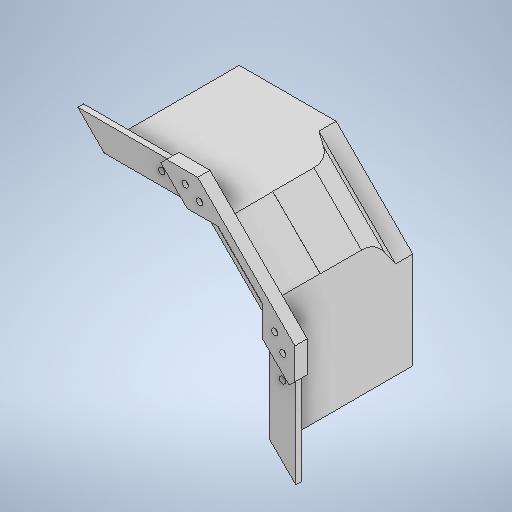
# Autodesk Inventor part: KimiBottomCover
Saved by Autodesk Inventor 2025.1 (Build 291241000, 241)
## iProperties
Created: 2026-05-07
Part Number: KimiBottomCover
Material: Generic
Document SubType Name: Modeling
Designer: User
Density: 1 g/cm^3
Appearance: Default
Author: User
## iProperties of the stored document KimiBottomCover_3DPrint.ipt
Created: 2026-05-07
Part Number: KimiBottomCover_3DPrint
Material: Generic
Document SubType Name: Modeling
Designer: User
Density: 1 g/cm^3
Appearance: Default
Author: User
Autodesk Inventor part; units mm, degrees
ref_plane "YZ Plane" through (0, 0, 0) normal (1, 0, 0) x (0, 1, 0)
ref_plane "XZ Plane" through (0, 0, 0) normal (0, 1, 0) x (-1, 0, 0)
ref_plane "XY Plane" through (0, 0, 0) normal (0, 0, 1) x (1, 0, 0)
sketch "Sketch1" plane through (0, 0, 0) normal (0, 0, 1) x (1, 0, 0)
  circle A0 centre (-3.4009, 1.926) radius 1.5 projected
  circle A1 centre (3.4009, -1.926) radius 1.5 projected
  circle A2 centre (38.7849, -37.31) radius 1.5 projected
  circle A3 centre (42.6369, -44.1118) radius 1.5 projected
  circle A4 centre (-3.4009, 1.926) radius 1.5 projected
  circle A5 centre (3.4009, -1.926) radius 1.5 projected
  line L0 (-12.5711, 5.5) -> (-1.5711, -5.5) projected
  line L1 (-1.5711, -5.5) -> (12.5711, -5.5) projected
  line L2 (12.5711, -5.5) -> (1.5711, 5.5) projected
  line L3 (1.5711, 5.5) -> (-12.5711, 5.5) projected
  circle A6 centre (38.7849, -37.31) radius 1.5 projected
  circle A7 centre (42.6369, -44.1118) radius 1.5 projected
  line L4 (46.2109, -53.282) -> (46.2109, -39.1398) projected
  line L5 (46.2109, -39.1398) -> (35.2109, -28.1398) projected
  line L6 (35.2109, -28.1398) -> (35.2109, -42.282) projected
  line L7 (35.2109, -42.282) -> (46.2109, -53.282) projected
  line L8 (35.1109, -27.8984) -> (46.3109, -39.0984)
  line L9 (46.3109, -39.0984) -> (46.3109, -53.5234)
  line L10 (46.3109, -53.5234) -> (35.1109, -42.3234)
  line L11 (35.1109, -42.3234) -> (35.1109, -27.8984)
  line L12 (12.8125, -5.6) -> (-1.6125, -5.6)
  line L13 (-1.6125, -5.6) -> (-12.8125, 5.6)
  line L14 (-12.8125, 5.6) -> (1.6125, 5.6)
  line L15 (1.6125, 5.6) -> (12.8125, -5.6)
  line L16 (-2.4409, -7.6) -> (17.6409, -7.6)
  line L17 (17.6409, -7.6) -> (2.4409, 7.6)
  line L18 (2.4409, 7.6) -> (-17.6409, 7.6)
  line L19 (-17.6409, 7.6) -> (-2.4409, -7.6)
  line L20 (33.1109, -43.1518) -> (48.3109, -58.3518)
  line L21 (48.3109, -58.3518) -> (48.3109, -38.27)
  line L22 (48.3109, -38.27) -> (33.1109, -23.07)
  line L23 (33.1109, -23.07) -> (33.1109, -43.1518)
  line L24 (46.3109, -53.5234) -> (44.8967, -54.9376)
  line L25 (44.8967, -54.9376) -> (45.6038, -55.6447)
  line L26 (45.6038, -55.6447) -> (48.3109, -52.9376)
  line L27 (-12.8125, 5.6) -> (-14.2267, 4.1858)
  line L28 (-14.2267, 4.1858) -> (-14.9338, 4.8929)
  line L29 (-14.9338, 4.8929) -> (-12.2267, 7.6)
  point P0 (0, 0)
  dimension "d0" = 0.1
  dimension "d1" = 0.1
  dimension "d2" = 2
  dimension "d3" = 2
  dimension "d4" = 1
  dimension "d5" = 1
  constraints: 44 end point, 6 point on line, 4 perpendicular, 12 other
  measures "d0" distance between parallel lines of L5 L8
  measures "d1" distance between parallel lines of L1 L12
  measures "d2" distance between parallel lines of L12 L16
  measures "d3" distance between parallel lines of L10 L20
  measures "d4" distance of L24.end L25.end
  measures "d5" distance of L27.end L28.end
ref_plane "Work Plane1" through (-57.7526, -5.5, -4) normal (0, 0, 1) x (1, 0, 0)
extrude "Extrusion1" add sketch "Sketch1" against normal up to surface (4 mm away) contours L19 L29 L18 L17 L16 | L23 L22 L21 L26 L20
sketch "Sketch2" plane through (0, 0, 0) normal (0, 0, 1) x (1, 0, 0)
  line L0 (-2.4409, -7.6) -> (17.6409, -7.6) projected
  line L1 (17.6409, -7.6) -> (2.4409, 7.6) projected
  line L2 (2.4409, 7.6) -> (-12.2267, 7.6) projected
  line L3 (-12.2267, 7.6) -> (-14.9338, 4.8929) projected
  line L4 (-14.9338, 4.8929) -> (-2.4409, -7.6) projected
  line L5 (-12.8125, 5.6) -> (1.6125, 5.6) projected
  line L6 (1.6125, 5.6) -> (12.8125, -5.6) projected
  line L7 (12.8125, -5.6) -> (-1.6125, -5.6) projected
  line L8 (-1.6125, -5.6) -> (-12.8125, 5.6) projected
  line L9 (45.6038, -55.6447) -> (48.3109, -52.9376) projected
  line L10 (48.3109, -52.9376) -> (48.3109, -38.27) projected
  line L11 (48.3109, -38.27) -> (33.1109, -23.07) projected
  line L12 (33.1109, -23.07) -> (33.1109, -43.1518) projected
  line L13 (33.1109, -43.1518) -> (45.6038, -55.6447) projected
  line L14 (46.3109, -53.5234) -> (35.1109, -42.3234) projected
  line L15 (35.1109, -42.3234) -> (35.1109, -27.8984) projected
  line L16 (35.1109, -27.8984) -> (46.3109, -39.0984) projected
  line L17 (46.3109, -39.0984) -> (46.3109, -53.5234) projected
  point P0 (0, 0)
extrude "Extrusion2" add sketch "Sketch2" along normal blind 1.8 contours L4 L3 L2 L1 L0 | L5 L6 L7 L8 | L13 L12 L11 L10 L9 | L14 L15 L16 L17
sketch "Sketch3" plane through (0, 0, 1.8) normal (0, 0, 1) x (1, 0, 0)
  circle A0 centre (-3.4009, 1.926) radius 1.5 projected
  circle A1 centre (3.4009, -1.926) radius 1.5 projected
  circle A2 centre (38.7849, -37.31) radius 1.5 projected
  circle A3 centre (42.6369, -44.1118) radius 1.5 projected
  point P0 (0, 0)
extrude "Extrusion3" cut sketch "Sketch3" against normal blind 1.8
sketch "Sketch4" plane through (17.6409, -7.6, -4) normal (0, 0, -1) x (-1, 0, 0)
  line L0 (19.2534, 2) -> (4.8284, 2) projected
  line L1 (-17.47, -20.2984) -> (-17.47, -34.7234) projected
  line L2 (-15.47, -35.5518) -> (-15.47, -15.47) projected
  line L3 (0, 0) -> (20.0818, 0) projected
  line L4 (69.8935, 7.6) -> (65.5651, 3.2716) projected
  line L5 (-18.7415, -81.0351) -> (-23.07, -85.3635) projected
  line L6 (-28.67, -31.4984) -> (-17.47, -20.2984) projected
  line L7 (-17.47, -20.2984) -> (4.8284, 2)
  line L8 (-30.67, -30.67) -> (-15.47, -15.47) projected
  line L9 (-17.47, -20.2984) -> (-17.47, -79.7635)
  line L10 (-17.47, -20.2984) -> (41.9951, -20.2984) construction
  line L11 (-15.47, -35.5518) -> (-27.9629, -48.0447) projected
  line L12 (-15.47, -35.5518) -> (-15.47, -77.7635)
  line L13 (-15.47, -77.7635) -> (-17.47, -79.7635)
  line L14 (4.8284, 2) -> (64.2935, 2)
  line L15 (20.0818, 0) -> (0, 0) projected
  line L16 (2.8284, 0) -> (62.2935, 0)
  line L17 (62.2935, 0) -> (64.2935, 2)
  line L18 (4.8284, 2) -> (6.2426, 0.5858)
  line L19 (6.2426, 0.5858) -> (-15.47, -21.1268)
  point P0 (17.6409, 7.6)
  point P1 (5.6569, 0)
  point P2 (19.2534, 2)
  point P3 (-17.47, -34.7234)
  point P4 (-17.47, -79.7635)
  dimension "d12" = 90
  dimension "d13" = 2
  constraints: 20 end point, 5 point on line, 3 perpendicular, 1 horizontal, 1 parallel, 1 vertical
  measures "d12" angle of L9 L10
  measures "d13" distance of L0.end L18.end
extrude "Extrusion4" add sketch "Sketch4" along normal blind 1.8
sketch "Sketch5" plane through (17.6409, -7.6, -4) normal (0, 0, 1) x (1, 0, 0)
  line L0 (15.47, -35.5518) -> (27.9629, -48.0447) projected
  line L1 (15.47, -77.7635) -> (15.47, -35.5518) projected
  line L2 (17.47, -79.7635) -> (15.47, -77.7635) projected
  line L3 (-20.0818, 0) -> (-62.2935, 0) projected
  line L4 (-32.5747, 12.4929) -> (-20.0818, 0) projected
  line L5 (-62.2935, 0) -> (-64.2935, 2) projected
  line L6 (-32.5747, 12.4929) -> (-74.7864, 12.4929)
  line L7 (-74.7864, 12.4929) -> (-62.2935, 0)
  line L8 (27.9629, -48.0447) -> (27.9629, -90.2564)
  line L9 (27.9629, -90.2564) -> (15.47, -77.7635)
  point P0 (-17.6409, 7.6)
  constraints: 8 end point, 1 collinear, 1 horizontal, 1 perpendicular, 1 point on line
extrude "Extrusion5" add sketch "Sketch5" along normal blind 2
sketch "Sketch6" plane through (17.6409, -7.6, -5.8) normal (0, 0, -1) x (-1, 0, 0)
  line L0 (5.6569, 0) -> (62.2935, 0) projected
  line L1 (62.2935, 0) -> (64.2935, 2) projected
  line L2 (64.2935, 2) -> (4.8284, 2) projected
  line L3 (4.8284, 2) -> (-17.47, -20.2984) projected
  line L4 (-17.47, -20.2984) -> (-17.47, -79.7635) projected
  line L5 (-17.47, -79.7635) -> (-15.47, -77.7635) projected
  line L6 (-15.47, -77.7635) -> (-15.47, -21.1268) projected
  line L7 (-15.47, -21.1268) -> (5.6569, 0) projected
  point P0 (17.6409, 7.6)
ref_plane "Work Plane2" through (-52.2526, -92.9635, -66.9376) normal (0, 0, -1) x (0, 1, 0)
extrude "Extrusion6" add sketch "Sketch6" along normal up to surface (61.1376 mm away)
sketch "Sketch7" plane through (12.8125, -5.6, -66.9376) normal (0, 0, -1) x (-1, 0, 0)
  line L0 (-20.2489, -31.2727) -> (8.9571, -2.0667) projected
  line L1 (-18.8347, -32.6869) -> (10.3713, -3.4809)
  line L2 (57.4651, -2) -> (0.8284, -2) projected
  line L3 (-20.2984, -23.1268) -> (-20.2984, -79.7635) projected
  line L4 (11.8522, -2) -> (-20.2984, -34.1506)
  line L5 (13.2664, -3.4142) -> (-18.8842, -35.5648)
  line L6 (-20.2984, -36.979) -> (14.6806, -2)
  point P0 (12.8125, 5.6)
  point P1 (10.3713, -3.4809)
  dimension "d20" = 2
  dimension "d21" = 2
  constraints: 8 end point, 6 point on line, 2 parallel
  measures "d20" distance between parallel lines of L0 L1
  measures "d21" distance between parallel lines of L4 L5
extrude "Extrusion7" add sketch "Sketch7" against normal blind 2
sketch "Sketch8" plane through (12.8125, -5.6, -64.9376) normal (0, 0, 1) x (1, 0, 0)
  line L0 (-14.6806, -2) -> (20.2984, -36.979) projected
  line L1 (20.2984, -34.1506) -> (-11.8522, -2) projected
  line L2 (2.8089, -19.4895) -> (4.2231, -18.0753)
  line L3 (3.516, -20.1966) -> (4.9302, -18.7824)
  line L4 (4.9302, -18.7824) -> (3.516, -17.3682)
  line L5 (3.516, -17.3682) -> (2.1018, -18.7824)
  line L6 (2.1018, -18.7824) -> (3.516, -20.1966)
  line L7 (3.516, -20.1966) -> (3.516, -17.3682) construction
  line L8 (4.9302, -18.7824) -> (2.1018, -18.7824) construction
  point P0 (-12.8125, 5.6)
  point P1 (3.516, -18.7824)
  point P2 (3.516, -20.1966)
  point P3 (3.516, -17.3682)
  point P4 (2.1018, -18.7824)
  dimension "d24" = 2
  constraints: 14 end point, 5 midpoint, 2 parallel, 2 perpendicular
  measures "d24" distance of L4.end L3.end
extrude "Extrusion8" add sketch "Sketch8" along normal blind 2
sketch "Sketch9" plane through (14.9143, -24.3824, -64.9376) normal (-0.7071068, 0.7071068, 0) x (-0.7071068, -0.7071068, 0)
  line L0 (-4.2088, 4.763) -> (-8.9478, 9.5057)
  line L1 (-7.5369, 1.0199) -> (-4.2089, 4.3453)
  line L2 (-4.2088, 4.763) -> (-4, 4.554)
  line L3 (-4, 4.554) -> (-4.2089, 4.3453)
  arc A0 (-14.215, 22.2357) -> (-8.9478, 9.5057) centre (3.785, 22.2287) ccw
  line L4 (-14.2133, 26.4375) -> (-14.215, 22.2357)
  line L5 (-14.2074, 41.6357) -> (-14.2133, 26.4375)
  arc A1 (-11.715, 22.2347) -> (-7.1794, 11.2728) centre (3.785, 22.2287) ccw
  line L6 (-11.715, 22.2347) -> (-11.7133, 26.4365)
  line L7 (-11.7133, 26.4365) -> (-11.7074, 41.6347)
  line L8 (0, 0) -> (0, 2)
  line L9 (-7.1794, 11.2728) -> (-2, 6.0894)
  line L10 (-2, 2) -> (-2, 6.0894)
  line L11 (0, 0) -> (-2, 0)
  line L12 (0, 0) -> (-14.2236, 0)
  line L13 (0, 0) -> (14.2236, 0) construction
  line L14 (-14.2236, 0) -> (-14.215, 22.2357)
  line L15 (-2, 0) -> (-2, 2)
  line L16 (-2, -2) -> (-2, 0)
  line L17 (-2, -2) -> (-14.2236, -2)
  line L18 (-2, -2) -> (10.2236, -2) construction
  line L19 (-14.2236, -2) -> (-14.2236, 0)
  line L20 (-14.2074, 41.6357) -> (-11.7074, 41.6347)
  line L21 (-14.2074, 41.6357) -> (-14.2066, 43.6357)
  line L22 (-14.2066, 43.6357) -> (-11.7074, 43.6347)
  line L23 (-11.7074, 43.6347) -> (-11.7074, 41.6347)
  line L24 (-11.795, 60.9376) -> (-11.795, -2)
  point P0 (-6.695, 64.9376)
extrude "Extrusion9" cut sketch "Sketch9" along normal through all both and the other way through all contours L4 L5 L20 L24 A0 | A0 L24 L12 L14 | L24 L20 L7 L6 A1 L9 L10 L15 L12 | L12 L24 L17 L19 | L12 L16 L17 L24
sketch "Sketch10" plane through (14.9143, -24.3824, -64.9376) normal (-0.7071068, 0.7071068, 0) x (-0.7071068, -0.7071068, 0)
  line L0 (0, 0) -> (-2, 0) projected
  line L1 (0, 0) -> (0, 2) projected
  line L2 (-2, 2) -> (0, 2) projected
  line L3 (-2, 0) -> (-2, 2) projected
  line L4 (-2, 6.0894) -> (-2, 0) projected
  line L5 (-7.1794, 11.2728) -> (-2, 6.0894) projected
  arc A0 (-9.795, 14.7566) -> (-7.1794, 11.2728) centre (3.785, 22.2287) ccw projected
  line L6 (-9.795, 60.9376) -> (-9.795, 14.7566) projected
  line L7 (0, 0) -> (0, 6.9174)
  line L8 (0, 6.9174) -> (-5.7646, 12.6865)
  arc A1 (-7.795, 15.2895) -> (-5.7646, 12.6865) centre (3.785, 22.2287) ccw
  line L9 (-7.795, 15.2895) -> (-7.795, 60.9376)
  line L10 (-9.795, 14.7566) -> (-9.795, 16.7566)
  line L11 (-9.795, 14.7566) -> (-7.795, 14.7566) construction
  line L12 (-9.795, 16.7566) -> (-7.795, 16.7566)
  point P0 (-6.695, 64.9376)
  point P1 (0, 0.0038)
  dimension "d34" = 2
  dimension "d35" = 2
  dimension "d36" = 90
  dimension "d37" = 90
  constraints: 12 end point, 2 point on circle, 2 point on line, 1 centre point, 1 horizontal, 1 perpendicular, 3 other
  measures "d34" radial gap between concentric circles of A0 A1
  measures "d35" distance of L6.end L10.end
  measures "d36" angle of L11 L10
  measures "d37" angle of L10 L12
extrude "Extrusion10" add sketch "Sketch10" along normal through all both and the other way through all
sketch "Sketch11" plane through (-1.0397, -5.6, -66.9376) normal (0, 0, -1) x (-1, 0, 0)
  line L0 (43.6129, -2) -> (0.8284, -2) projected
  line L1 (-34.1506, -36.979) -> (0.8284, -2) projected
  line L2 (-34.1506, -36.979) -> (-34.1506, -79.7635) projected
  line L3 (43.6129, -2) -> (-34.1506, -79.7635)
  point P0 (-1.0397, 5.6)
  constraints: 2 end point
extrude "Extrusion11" add sketch "Sketch11" against normal blind 2
sketch "Sketch14" plane through (-1.0397, -5.6, -64.9376) normal (0, 0, 1) x (1, 0, 0)
  line L0 (-43.6129, -2) -> (34.1506, -79.7635) projected
  line L1 (34.1506, -36.979) -> (34.1506, -79.7635) projected
  line L2 (-0.8284, -2) -> (34.1506, -36.979) projected
  line L3 (-43.6129, -2) -> (-0.8284, -2) projected
  line L4 (32.1506, -74.9351) -> (-38.7845, -4)
  line L5 (-38.7845, -4) -> (-1.6569, -4)
  line L6 (-1.6569, -4) -> (32.1506, -37.8075)
  line L7 (32.1506, -37.8075) -> (32.1506, -74.9351)
  line L8 (-38.7845, -4) -> (-40.7845, -2)
  line L9 (32.1506, -74.9351) -> (34.1506, -76.9351)
  point P0 (1.0397, 5.6)
  dimension "d42" = 2
  constraints: 12 end point, 3 point on line, 1 parallel, 3 other
  measures "d42" distance between parallel lines of L0 L4
extrude "Extrusion12" add sketch "Sketch14" along normal blind 40 contours L3 L8 L4 L9 L1 L0
chamfer "Chamfer1" distance 2 angle 45 2 edges at (-41.8242, -7.6, -44.9376) (33.1109, -82.5351, -44.9376)
sketch "Sketch15" plane through (17.6409, -7.6, -4) normal (0, 0, 1) x (1, 0, 0)
  line L0 (-20.0818, 0) -> (0, 0) projected
  line L1 (15.47, -21.1268) -> (-5.6569, 0) projected
  line L2 (15.47, -15.47) -> (15.47, -35.5518) projected
  line L3 (0, 0) -> (15.47, -15.47)
  point P0 (-17.6409, 7.6)
  constraints: 2 end point
extrude "Extrusion13" add sketch "Sketch15" along normal up to surface (5.8 mm away)
sketch "Sketch16" plane through (17.6409, -7.6, -2) normal (0, 0, 1) x (1, 0, 0)
  line L0 (-32.5747, 12.4929) -> (-20.0818, 0) projected
  line L1 (-32.5747, 12.4929) -> (-74.7864, 12.4929) projected
  line L2 (-74.7864, 12.4929) -> (-62.2935, 0) projected
  line L3 (-62.2935, 0) -> (-20.0818, 0) projected
  line L4 (15.47, -35.5518) -> (27.9629, -48.0447) projected
  line L5 (15.47, -35.5518) -> (15.47, -77.7635) projected
  line L6 (15.47, -77.7635) -> (27.9629, -90.2564) projected
  line L7 (27.9629, -90.2564) -> (27.9629, -48.0447) projected
  point P0 (-17.6409, 7.6)
extrude "Extrusion14" add sketch "Sketch16" along normal blind 0.7
sketch "Sketch17" plane through (17.6409, -7.6, -1.3) normal (0, 0, 1) x (1, 0, 0)
  line L0 (-32.5747, 12.4929) -> (-74.7864, 12.4929) projected
  line L1 (-62.2935, 0) -> (-20.0818, 0) projected
  line L2 (15.47, -35.5518) -> (15.47, -77.7635) projected
  line L3 (27.9629, -90.2564) -> (27.9629, -48.0447) projected
  line L4 (15.47, -35.5518) -> (27.9629, -48.0447) projected
  line L5 (-32.5747, 12.4929) -> (-20.0818, 0) projected
  circle A0 centre (-35.1621, 6.2464) radius 6.2464
  circle A1 centre (21.7164, -50.6321) radius 6.2464
  circle A2 centre (21.7164, -50.6321) radius 1.5
  circle A3 centre (-35.1621, 6.2464) radius 1.5
  point P0 (-17.6409, 7.6)
  dimension "d52" = 3
  dimension "d53" = 3
  constraints: 6 tangent, 4 centre point, 2 coincident
  measures "d52" diameter of A2
  measures "d53" diameter of A3
extrude "Extrusion15" cut sketch "Sketch17" against normal through all contours A2 | A3
sketch "Sketch18" plane through (-46.6526, -5.6, -4) normal (-0.7071068, -0.7071068, 0) x (-0.7071068, 0.7071068, 0)
  line L0 (-1.7022, 32.5311) -> (-114.1155, 32.5311) construction
  line L1 (-114.1155, 32.5311) -> (-114.1155, 43.7799) construction
  line L2 (-114.1155, 43.7799) -> (-1.7022, 43.7799) construction
  line L3 (-1.7022, 43.7799) -> (-1.7022, 32.5311) construction
  spline S0 degree 2 poles (-6.1526, 35.0507) (-7.0471, 35.0507) (-8.3069, 35.4682) (-8.6871, 35.8335) knots 0 0 0 1 2 2 2
  spline S1 degree 2 poles (-8.6871, 35.8335) (-9.0598, 36.1838) (-9.3952, 37.1082) (-9.3952, 37.5927) knots 0 0 0 1 2 2 2
  spline S2 degree 2 poles (-9.3952, 37.5927) (-9.3952, 38.5692) (-8.5902, 40.1347) (-7.8969, 40.7683) knots 0 0 0 1 2 2 2
  spline S3 degree 2 poles (-7.8969, 40.7683) (-7.1962, 41.4169) (-5.2953, 42.535) (-4.2069, 43.0643) knots 0 0 0 1 2 2 2
  line L4 (-4.2069, 43.0643) -> (-4.2069, 40.7758)
  spline S4 degree 2 poles (-4.2069, 40.7758) (-4.8033, 40.5) (-5.9438, 39.844) (-6.3986, 39.4638) knots 0 0 0 1 2 2 2
  spline S5 degree 2 poles (-6.3986, 39.4638) (-6.8831, 39.0612) (-7.3676, 38.3083) (-7.3676, 37.9505) knots 0 0 0 1 2 2 2
  spline S6 degree 2 poles (-7.3676, 37.9505) (-7.3676, 37.7791) (-7.2558, 37.5256) (-7.1216, 37.4362) knots 0 0 0 1 2 2 2
  spline S7 degree 2 poles (-7.1216, 37.4362) (-6.9576, 37.3393) (-6.5626, 37.2722) (-6.2346, 37.2722) knots 0 0 0 1 2 2 2
  line L5 (-6.2346, 37.2722) -> (-2.1793, 37.2722)
  line L6 (-2.1793, 37.2722) -> (-2.1793, 32.5311)
  line L7 (-2.1793, 32.5311) -> (-4.2069, 32.5311)
  line L8 (-4.2069, 32.5311) -> (-4.2069, 35.0507)
  line L9 (-4.2069, 35.0507) -> (-6.1526, 35.0507)
  line L10 (-13.4728, 35.0507) -> (-15.5303, 38.0698)
  spline S8 degree 2 poles (-15.5303, 38.0698) (-16.1043, 37.7344) (-16.6335, 36.6684) (-16.6335, 35.908) knots 0 0 0 1 2 2 2
  line L11 (-16.6335, 35.908) -> (-16.6335, 35.0507)
  line L12 (-16.6335, 35.0507) -> (-18.6611, 35.0507)
  line L13 (-18.6611, 35.0507) -> (-18.6611, 35.908)
  spline S9 degree 2 poles (-18.6611, 35.908) (-18.6611, 37.1007) (-17.5504, 38.7705) (-16.3726, 39.3147) knots 0 0 0 1 2 2 2
  line L14 (-16.3726, 39.3147) -> (-18.8028, 42.8705)
  line L15 (-18.8028, 42.8705) -> (-16.1117, 42.8705)
  line L16 (-16.1117, 42.8705) -> (-13.6145, 39.2103)
  spline S10 degree 2 poles (-13.6145, 39.2103) (-13.279, 39.5011) (-12.9137, 40.4552) (-12.9137, 41.0963) knots 0 0 0 1 2 2 2
  line L17 (-12.9137, 41.0963) -> (-12.9137, 42.8705)
  line L18 (-12.9137, 42.8705) -> (-10.8861, 42.8705)
  line L19 (-10.8861, 42.8705) -> (-10.8861, 41.0963)
  spline S11 degree 2 poles (-10.8861, 41.0963) (-10.8861, 40.1198) (-11.7658, 38.4798) (-12.6976, 37.8611) knots 0 0 0 1 2 2 2
  line L20 (-12.6976, 37.8611) -> (-10.7818, 35.0507)
  line L21 (-10.7818, 35.0507) -> (-13.4728, 35.0507)
  line L22 (-26.8983, 42.8705) -> (-24.8707, 42.8705)
  line L23 (-24.8707, 42.8705) -> (-24.8707, 38.7482)
  spline S12 degree 2 poles (-24.8707, 38.7482) (-24.8707, 38.3605) (-24.7216, 37.7344) (-24.4682, 37.5182) knots 0 0 0 1 2 2 2
  spline S13 degree 2 poles (-24.4682, 37.5182) (-24.2147, 37.302) (-23.2829, 37.0784) (-22.5076, 37.0784) knots 0 0 0 1 2 2 2
  spline S14 degree 2 poles (-22.5076, 37.0784) (-21.9038, 37.0784) (-20.5247, 37.2051) (-19.9806, 37.2722) knots 0 0 0 1 2 2 2
  line L24 (-19.9806, 37.2722) -> (-19.9135, 37.2722)
  line L25 (-19.9135, 37.2722) -> (-19.9135, 35.0358)
  spline S15 degree 2 poles (-19.9135, 35.0358) (-20.3757, 34.9762) (-21.9187, 34.8569) (-22.5375, 34.8569) knots 0 0 0 1 2 2 2
  spline S16 degree 2 poles (-22.5375, 34.8569) (-23.8569, 34.8569) (-25.5118, 35.3117) (-26.0187, 35.7813) knots 0 0 0 1 2 2 2
  spline S17 degree 2 poles (-26.0187, 35.7813) (-26.5032, 36.2509) (-26.8983, 37.6524) (-26.8983, 38.614) knots 0 0 0 1 2 2 2
  line L26 (-26.8983, 38.614) -> (-26.8983, 42.8705)
  line L27 (-30.797, 39.3072) -> (-30.797, 40.649)
  line L28 (-30.797, 40.649) -> (-31.1772, 40.649)
  spline S18 degree 2 poles (-31.1772, 40.649) (-32.1015, 40.649) (-33.3539, 40.3434) (-33.8235, 40.0005) knots 0 0 0 1 2 2 2
  spline S19 degree 2 poles (-33.8235, 40.0005) (-34.7702, 39.3221) (-35.8884, 36.8025) (-36.2387, 35.0507) knots 0 0 0 1 2 2 2
  line L29 (-36.2387, 35.0507) -> (-38.2738, 35.0507)
  spline S20 degree 2 poles (-38.2738, 35.0507) (-37.7967, 37.5629) (-35.9555, 41.1261) (-34.6435, 42.0207) knots 0 0 0 1 2 2 2
  spline S21 degree 2 poles (-34.6435, 42.0207) (-33.98, 42.453) (-32.2879, 42.8705) (-31.1623, 42.8705) knots 0 0 0 1 2 2 2
  line L30 (-31.1623, 42.8705) -> (-28.7694, 42.8705)
  line L31 (-28.7694, 42.8705) -> (-28.7694, 35.0507)
  line L32 (-28.7694, 35.0507) -> (-30.797, 35.0507)
  line L33 (-30.797, 35.0507) -> (-30.797, 37.5331)
  spline S22 degree 2 poles (-30.797, 37.5331) (-31.1101, 37.5331) (-31.5573, 37.3989) (-31.7661, 37.2274) knots 0 0 0 1 2 2 2
  spline S23 degree 2 poles (-31.7661, 37.2274) (-32.1015, 36.9665) (-32.5041, 35.9155) (-32.6382, 35.0507) knots 0 0 0 1 2 2 2
  line L34 (-32.6382, 35.0507) -> (-34.6733, 35.0507)
  spline S24 degree 2 poles (-34.6733, 35.0507) (-34.39, 36.5342) (-33.4731, 38.2785) (-32.9588, 38.6736) knots 0 0 0 1 2 2 2
  spline S25 degree 2 poles (-32.9588, 38.6736) (-32.4742, 39.0314) (-31.4083, 39.3072) (-30.797, 39.3072) knots 0 0 0 1 2 2 2
  line L35 (-42.2396, 39.4638) -> (-40.212, 39.4638)
  line L36 (-40.212, 39.4638) -> (-40.212, 37.4958)
  spline S26 degree 2 poles (-40.212, 37.4958) (-40.212, 37.3094) (-39.9362, 37.0784) (-39.72, 37.0784) knots 0 0 0 1 2 2 2
  spline S27 degree 2 poles (-39.72, 37.0784) (-39.3771, 37.0784) (-38.9298, 37.1231) (-38.736, 37.1529) knots 0 0 0 1 2 2 2
  line L37 (-38.736, 37.1529) -> (-38.736, 34.9315)
  spline S28 degree 2 poles (-38.736, 34.9315) (-38.9149, 34.9091) (-39.6529, 34.8569) (-40.0107, 34.8569) knots 0 0 0 1 2 2 2
  spline S29 degree 2 poles (-40.0107, 34.8569) (-41.0394, 34.8569) (-42.2396, 35.99) (-42.2396, 36.8175) knots 0 0 0 1 2 2 2
  line L38 (-42.2396, 36.8175) -> (-42.2396, 39.4638)
  line L39 (-55.4191, 42.8705) -> (-47.6292, 42.8705)
  line L40 (-47.6292, 42.8705) -> (-47.6292, 34.8569)
  line L41 (-47.6292, 34.8569) -> (-51.0582, 34.8569)
  spline S30 degree 2 poles (-51.0582, 34.8569) (-52.3851, 34.8569) (-54.04, 35.3117) (-54.5394, 35.7813) knots 0 0 0 1 2 2 2
  spline S31 degree 2 poles (-54.5394, 35.7813) (-55.024, 36.2509) (-55.4191, 37.6524) (-55.4191, 38.614) knots 0 0 0 1 2 2 2
  line L42 (-55.4191, 38.614) -> (-55.4191, 42.8705)
  line L43 (-53.3915, 40.7087) -> (-53.3915, 38.6885)
  spline S32 degree 2 poles (-53.3915, 38.6885) (-53.3915, 38.3009) (-53.2424, 37.6747) (-52.9889, 37.4585) knots 0 0 0 1 2 2 2
  spline S33 degree 2 poles (-52.9889, 37.4585) (-52.7355, 37.2424) (-51.8111, 37.0187) (-51.0284, 37.0187) knots 0 0 0 1 2 2 2
  line L44 (-51.0284, 37.0187) -> (-49.6568, 37.0187)
  line L45 (-49.6568, 37.0187) -> (-49.6568, 40.7087)
  line L46 (-49.6568, 40.7087) -> (-53.3915, 40.7087)
  spline S34 degree 2 poles (-60.9801, 40.2614) (-61.3752, 39.9185) (-62.0461, 39.0389) (-62.2697, 38.4425) knots 0 0 0 1 2 2 2
  spline S35 degree 2 poles (-62.2697, 38.4425) (-62.5083, 37.8163) (-62.7692, 36.2211) (-62.7692, 35.0507) knots 0 0 0 1 2 2 2
  line L47 (-62.7692, 35.0507) -> (-64.7968, 35.0507)
  spline S36 degree 2 poles (-64.7968, 35.0507) (-64.7968, 36.6162) (-64.3719, 38.8749) (-64.0215, 39.6576) knots 0 0 0 1 2 2 2
  spline S37 degree 2 poles (-64.0215, 39.6576) (-63.6637, 40.4478) (-62.7468, 41.5287) (-62.2623, 41.9014) knots 0 0 0 1 2 2 2
  spline S38 degree 2 poles (-62.2623, 41.9014) (-61.241, 42.7139) (-58.4828, 43.5936) (-56.6416, 43.7799) knots 0 0 0 1 2 2 2
  line L48 (-56.6416, 43.7799) -> (-56.6416, 41.5585)
  spline S39 degree 2 poles (-56.6416, 41.5585) (-57.4467, 41.4989) (-58.7288, 41.2976) (-59.2432, 41.141) knots 0 0 0 1 2 2 2
  line L49 (-59.2432, 41.141) -> (-57.238, 35.0507)
  line L50 (-57.238, 35.0507) -> (-59.3699, 35.0507)
  line L51 (-59.3699, 35.0507) -> (-60.9801, 40.2614)
  spline S40 degree 2 poles (-73.7048, 35.0507) (-74.5994, 35.0507) (-75.8592, 35.4682) (-76.2394, 35.8335) knots 0 0 0 1 2 2 2
  spline S41 degree 2 poles (-76.2394, 35.8335) (-76.6121, 36.1838) (-76.9475, 37.1082) (-76.9475, 37.5927) knots 0 0 0 1 2 2 2
  spline S42 degree 2 poles (-76.9475, 37.5927) (-76.9475, 38.5692) (-76.1425, 40.1347) (-75.4492, 40.7683) knots 0 0 0 1 2 2 2
  spline S43 degree 2 poles (-75.4492, 40.7683) (-74.7485, 41.4169) (-72.8476, 42.535) (-71.7592, 43.0643) knots 0 0 0 1 2 2 2
  line L52 (-71.7592, 43.0643) -> (-71.7592, 40.7758)
  spline S44 degree 2 poles (-71.7592, 40.7758) (-72.3556, 40.5) (-73.4961, 39.844) (-73.9508, 39.4638) knots 0 0 0 1 2 2 2
  spline S45 degree 2 poles (-73.9508, 39.4638) (-74.4354, 39.0612) (-74.9199, 38.3083) (-74.9199, 37.9505) knots 0 0 0 1 2 2 2
  spline S46 degree 2 poles (-74.9199, 37.9505) (-74.9199, 37.7791) (-74.8081, 37.5256) (-74.6739, 37.4362) knots 0 0 0 1 2 2 2
  spline S47 degree 2 poles (-74.6739, 37.4362) (-74.5099, 37.3393) (-74.1148, 37.2722) (-73.7868, 37.2722) knots 0 0 0 1 2 2 2
  line L53 (-73.7868, 37.2722) -> (-69.7316, 37.2722)
  line L54 (-69.7316, 37.2722) -> (-69.7316, 32.5311)
  line L55 (-69.7316, 32.5311) -> (-71.7592, 32.5311)
  line L56 (-71.7592, 32.5311) -> (-71.7592, 35.0507)
  line L57 (-71.7592, 35.0507) -> (-73.7048, 35.0507)
  spline S48 degree 2 poles (-81.3233, 38.1294) (-81.0251, 38.1294) (-80.6822, 38.5543) (-80.6822, 38.9569) knots 0 0 0 1 2 2 2
  line L58 (-80.6822, 38.9569) -> (-80.6822, 42.8705)
  line L59 (-80.6822, 42.8705) -> (-78.6546, 42.8705)
  line L60 (-78.6546, 42.8705) -> (-78.6546, 38.9345)
  spline S49 degree 2 poles (-78.6546, 38.9345) (-78.6546, 38.6214) (-78.8559, 38.1071) (-79.0199, 37.9282) knots 0 0 0 1 2 2 2
  spline S50 degree 2 poles (-79.0199, 37.9282) (-79.1615, 37.7567) (-79.5715, 37.5629) (-79.7206, 37.5405) knots 0 0 0 1 2 2 2
  line L61 (-79.7206, 37.5405) -> (-77.8644, 36.9293)
  line L62 (-77.8644, 36.9293) -> (-77.8644, 34.6109)
  line L63 (-77.8644, 34.6109) -> (-81.9718, 35.9602)
  line L64 (-81.9718, 35.9602) -> (-81.9718, 38.2785)
  spline S51 degree 2 poles (-81.9718, 38.2785) (-81.8004, 38.2189) (-81.4575, 38.1294) (-81.3233, 38.1294) knots 0 0 0 1 2 2 2
  line L65 (-85.7662, 35.0507) -> (-87.8236, 38.0698)
  spline S52 degree 2 poles (-87.8236, 38.0698) (-88.3976, 37.7344) (-88.9268, 36.6684) (-88.9268, 35.908) knots 0 0 0 1 2 2 2
  line L66 (-88.9268, 35.908) -> (-88.9268, 35.0507)
  line L67 (-88.9268, 35.0507) -> (-90.9545, 35.0507)
  line L68 (-90.9545, 35.0507) -> (-90.9545, 35.908)
  spline S53 degree 2 poles (-90.9545, 35.908) (-90.9545, 37.1007) (-89.8437, 38.7705) (-88.6659, 39.3147) knots 0 0 0 1 2 2 2
  line L69 (-88.6659, 39.3147) -> (-91.0961, 42.8705)
  line L70 (-91.0961, 42.8705) -> (-88.405, 42.8705)
  line L71 (-88.405, 42.8705) -> (-85.9078, 39.2103)
  spline S54 degree 2 poles (-85.9078, 39.2103) (-85.5723, 39.5011) (-85.2071, 40.4552) (-85.2071, 41.0963) knots 0 0 0 1 2 2 2
  line L72 (-85.2071, 41.0963) -> (-85.2071, 42.8705)
  line L73 (-85.2071, 42.8705) -> (-83.1795, 42.8705)
  line L74 (-83.1795, 42.8705) -> (-83.1795, 41.0963)
  spline S55 degree 2 poles (-83.1795, 41.0963) (-83.1795, 40.1198) (-84.0591, 38.4798) (-84.9909, 37.8611) knots 0 0 0 1 2 2 2
  line L75 (-84.9909, 37.8611) -> (-83.0751, 35.0507)
  line L76 (-83.0751, 35.0507) -> (-85.7662, 35.0507)
  spline S56 degree 2 poles (-95.7253, 38.1294) (-95.4271, 38.1294) (-95.0842, 38.5543) (-95.0842, 38.9569) knots 0 0 0 1 2 2 2
  line L77 (-95.0842, 38.9569) -> (-95.0842, 42.8705)
  line L78 (-95.0842, 42.8705) -> (-93.0566, 42.8705)
  line L79 (-93.0566, 42.8705) -> (-93.0566, 38.9345)
  spline S57 degree 2 poles (-93.0566, 38.9345) (-93.0566, 38.6214) (-93.2579, 38.1071) (-93.4219, 37.9282) knots 0 0 0 1 2 2 2
  spline S58 degree 2 poles (-93.4219, 37.9282) (-93.5635, 37.7567) (-93.9735, 37.5629) (-94.1226, 37.5405) knots 0 0 0 1 2 2 2
  line L80 (-94.1226, 37.5405) -> (-92.2664, 36.9293)
  line L81 (-92.2664, 36.9293) -> (-92.2664, 34.6109)
  line L82 (-92.2664, 34.6109) -> (-96.3739, 35.9602)
  line L83 (-96.3739, 35.9602) -> (-96.3739, 38.2785)
  spline S59 degree 2 poles (-96.3739, 38.2785) (-96.2024, 38.2189) (-95.8595, 38.1294) (-95.7253, 38.1294) knots 0 0 0 1 2 2 2
  spline S60 degree 2 poles (-101.2938, 40.2614) (-101.6889, 39.9185) (-102.3598, 39.0389) (-102.5834, 38.4425) knots 0 0 0 1 2 2 2
  spline S61 degree 2 poles (-102.5834, 38.4425) (-102.822, 37.8163) (-103.0829, 36.2211) (-103.0829, 35.0507) knots 0 0 0 1 2 2 2
  line L84 (-103.0829, 35.0507) -> (-105.1105, 35.0507)
  spline S62 degree 2 poles (-105.1105, 35.0507) (-105.1105, 36.6162) (-104.6856, 38.8749) (-104.3352, 39.6576) knots 0 0 0 1 2 2 2
  spline S63 degree 2 poles (-104.3352, 39.6576) (-103.9774, 40.4478) (-103.0605, 41.5287) (-102.576, 41.9014) knots 0 0 0 1 2 2 2
  spline S64 degree 2 poles (-102.576, 41.9014) (-101.5547, 42.7139) (-98.7966, 43.5936) (-96.9553, 43.7799) knots 0 0 0 1 2 2 2
  line L85 (-96.9553, 43.7799) -> (-96.9553, 41.5585)
  spline S65 degree 2 poles (-96.9553, 41.5585) (-97.7604, 41.4989) (-99.0425, 41.2976) (-99.5569, 41.141) knots 0 0 0 1 2 2 2
  line L86 (-99.5569, 41.141) -> (-97.5517, 35.0507)
  line L87 (-97.5517, 35.0507) -> (-99.6836, 35.0507)
  line L88 (-99.6836, 35.0507) -> (-101.2938, 40.2614)
  spline S66 degree 2 poles (-110.3137, 35.0507) (-111.2082, 35.0507) (-112.468, 35.4682) (-112.8482, 35.8335) knots 0 0 0 1 2 2 2
  spline S67 degree 2 poles (-112.8482, 35.8335) (-113.2209, 36.1838) (-113.5564, 37.1082) (-113.5564, 37.5927) knots 0 0 0 1 2 2 2
  spline S68 degree 2 poles (-113.5564, 37.5927) (-113.5564, 38.5692) (-112.7513, 40.1347) (-112.058, 40.7683) knots 0 0 0 1 2 2 2
  spline S69 degree 2 poles (-112.058, 40.7683) (-111.3573, 41.4169) (-109.4564, 42.535) (-108.3681, 43.0643) knots 0 0 0 1 2 2 2
  line L89 (-108.3681, 43.0643) -> (-108.3681, 40.7758)
  spline S70 degree 2 poles (-108.3681, 40.7758) (-108.9644, 40.5) (-110.105, 39.844) (-110.5597, 39.4638) knots 0 0 0 1 2 2 2
  spline S71 degree 2 poles (-110.5597, 39.4638) (-111.0442, 39.0612) (-111.5288, 38.3083) (-111.5288, 37.9505) knots 0 0 0 1 2 2 2
  spline S72 degree 2 poles (-111.5288, 37.9505) (-111.5288, 37.7791) (-111.4169, 37.5256) (-111.2828, 37.4362) knots 0 0 0 1 2 2 2
  spline S73 degree 2 poles (-111.2828, 37.4362) (-111.1188, 37.3393) (-110.7237, 37.2722) (-110.3957, 37.2722) knots 0 0 0 1 2 2 2
  line L90 (-110.3957, 37.2722) -> (-106.3405, 37.2722)
  line L91 (-106.3405, 37.2722) -> (-106.3405, 32.5311)
  line L92 (-106.3405, 32.5311) -> (-108.3681, 32.5311)
  line L93 (-108.3681, 32.5311) -> (-108.3681, 35.0507)
  line L94 (-108.3681, 35.0507) -> (-110.3137, 35.0507)
  point P0 (-29.0286, -4)
  constraints: 2 other
emboss "Emboss1" sketch "Sketch18" operation cut depth 0.5 direction (0.7071068, 0.7071068, 0)
body "Solid1"
